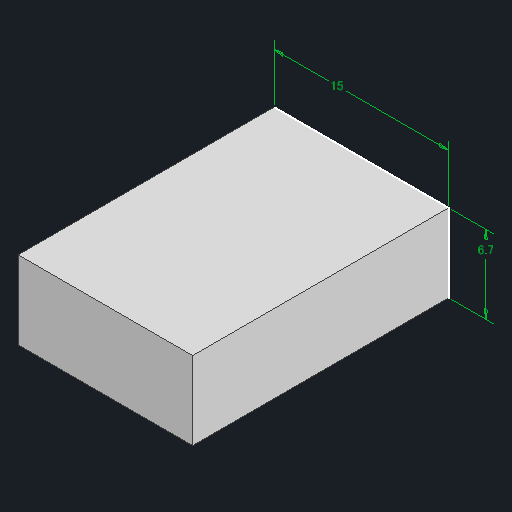
# Autodesk Inventor part: Lipo-1C-FX100C
Saved by Autodesk Inventor 2023.5 (Build 275446000, 446)
## iProperties
Created: 2025-01-19
Part Number: Lipo-1C-FX100C
Material: 一般
Document SubType Name: Modeling
Designer: IshiiLabHonda
Density: 1 g/cm^3
Appearance: 既定
Author: IshiiLabHonda
Autodesk Inventor part; units mm, degrees
ref_plane "YZ Plane" through (0, 0, 0) normal (1, 0, 0) x (0, 1, 0)
ref_plane "XZ Plane" through (0, 0, 0) normal (0, 1, 0) x (-1, 0, 0)
ref_plane "XY Plane" through (0, 0, 0) normal (0, 0, 1) x (1, 0, 0)
sketch "スケッチ1" plane through (0, 0, 0) normal (0, 0, 1) x (1, 0, 0)
  line L0 (-7.5, 3.35) -> (7.5, 3.35)
  line L1 (7.5, 3.35) -> (7.5, -3.35)
  line L2 (7.5, -3.35) -> (-7.5, -3.35)
  line L3 (-7.5, -3.35) -> (-7.5, 3.35)
  line L4 (-7.5, 3.35) -> (7.5, -3.35) construction
  line L5 (7.5, 3.35) -> (-7.5, -3.35) construction
  point P0 (0, 0)
  dimension "d0" = 15
  dimension "d1" = 6.7
  constraints: 12 end point, 2 midpoint, 2 parallel, 1 horizontal, 1 perpendicular
  measures "d0" distance of L0.start L0.end
  measures "d1" distance of L0.end L1.end
extrude "押し出し1" add sketch "スケッチ1" along normal blind 22
